Autodesk Fusion 360 part; units mm, degrees
(part 5 of 5)
  line L479 (14.0888, 19.1801) -> (13.1993, 20.0782)
  spline S498 degree 3 poles (13.1993, 20.0782) (12.7098, 20.5721) (12.0642, 21.2311) (11.7643, 21.5427) knots 0 0 0 0 1 1 1 1
  spline S499 degree 3 poles (11.7643, 21.5427) (11.0509, 22.2836) (10.6839, 22.4136) (10.1068, 22.1302) knots 0 0 0 0 1 1 1 1
  spline S500 degree 3 poles (10.1068, 22.1302) (9.2919, 21.7302) (9.2967, 20.4435) (10.115, 20.0204) knots 0 0 0 0 1 1 1 1
  spline S501 degree 3 poles (10.115, 20.0204) (10.2289, 19.9616) (10.2292, 19.9609) (10.2292, 19.6142) knots 0 0 0 0 1 1 1 1
  line L480 (10.2292, 19.6142) -> (10.2292, 19.2671)
  line L481 (10.2292, 19.2671) -> (10.124, 19.2919)
  spline S502 degree 3 poles (10.124, 19.2919) (9.1475, 19.5213) (8.5366, 20.6684) (8.8609, 21.6642) knots 0 0 0 0 1 1 1 1
  spline S503 degree 3 poles (8.7977, 26.7455) (8.8953, 27.5059) (9.4553, 28.1595) (10.2653, 28.4591) knots 0 0 0 0 1 1 1 1
  spline S504 degree 3 poles (10.2653, 28.4591) (10.5632, 28.5691) (12.2025, 28.6032) (12.6135, 28.5076) knots 0 0 0 0 1 1 1 1
  spline S505 degree 3 poles (12.6135, 28.5076) (14.8462, 27.9885) (14.8204, 24.7336) (12.5795, 24.2631) knots 0 0 0 0 1 1 1 1
  spline S506 degree 3 poles (12.5795, 24.2631) (12.2114, 24.1857) (10.8463, 24.1854) (10.4824, 24.2624) knots 0 0 0 0 1 1 1 1
  spline S507 degree 3 poles (10.4824, 24.2624) (9.5743, 24.455) (8.8991, 25.1822) (8.7787, 26.0974) knots 0 0 0 0 1 1 1 1
  spline S508 degree 3 poles (8.7787, 26.0974) (8.7488, 26.3241) (8.7505, 26.376) (8.7977, 26.7455) knots 0 0 0 0 1 1 1 1
  spline S509 degree 3 poles (8.8609, 32.4032) (9.1953, 33.4296) (10.3726, 33.9445) (11.3178, 33.4774) knots 0 0 0 0 1 1 1 1
  spline S510 degree 3 poles (11.3178, 33.4774) (11.5782, 33.3484) (11.7144, 33.2339) (12.4391, 32.5326) knots 0 0 0 0 1 1 1 1
  spline S511 degree 3 poles (12.4391, 32.5326) (13.0246, 31.9664) (13.2898, 31.7346) (13.352, 31.7346) knots 0 0 0 0 1 1 1 1
  line L482 (13.352, 31.7346) -> (13.4394, 31.7346)
  line L483 (13.4394, 31.7346) -> (13.4394, 32.6897)
  line L484 (13.4394, 32.6897) -> (13.4394, 33.6453)
  line L485 (13.4394, 33.6453) -> (13.7641, 33.6453)
  line L486 (13.7641, 33.6453) -> (14.0891, 33.6453)
  line L487 (14.0891, 33.6453) -> (14.0888, 31.782)
  line L488 (14.0888, 31.782) -> (14.0888, 29.9192)
  line L489 (14.0888, 29.9192) -> (13.2182, 30.798)
  spline S512 degree 3 poles (13.2182, 30.798) (12.7398, 31.2816) (12.0938, 31.9406) (11.7829, 32.2629) knots 0 0 0 0 1 1 1 1
  spline S513 degree 3 poles (11.7829, 32.2629) (11.0485, 33.0244) (10.6881, 33.1548) (10.1068, 32.8693) knots 0 0 0 0 1 1 1 1
  spline S514 degree 3 poles (10.1068, 32.8693) (9.2919, 32.4696) (9.2967, 31.1825) (10.115, 30.7594) knots 0 0 0 0 1 1 1 1
  spline S515 degree 3 poles (10.115, 30.7594) (10.2289, 30.7006) (10.2292, 30.7003) (10.2292, 30.3536) knots 0 0 0 0 1 1 1 1
  line L490 (10.2292, 30.3536) -> (10.2292, 30.0062)
  line L491 (10.2292, 30.0062) -> (10.124, 30.0309)
  spline S516 degree 3 poles (10.124, 30.0309) (9.1502, 30.2583) (8.5373, 31.4095) (8.8609, 32.4032) knots 0 0 0 0 1 1 1 1
  spline S517 degree 3 poles (8.8541, 37.2252) (9.1798, 38.1762) (10.3131, 38.4655) (10.9852, 37.769) knots 0 0 0 0 1 1 1 1
  spline S518 degree 3 poles (10.9852, 37.769) (11.2074, 37.5389) (11.2642, 37.5365) (11.4121, 37.7514) knots 0 0 0 0 1 1 1 1
  spline S519 degree 3 poles (11.4121, 37.7514) (12.1451, 38.8167) (13.8064, 38.4858) (14.2081, 37.1949) knots 0 0 0 0 1 1 1 1
  spline S520 degree 3 poles (14.2081, 37.1949) (14.5301, 36.1603) (13.9237, 35.1267) (12.855, 34.8897) knots 0 0 0 0 1 1 1 1
  line L492 (12.855, 34.8897) -> (12.7484, 34.866)
  line L493 (12.7484, 34.866) -> (12.7594, 35.1993)
  line L494 (12.7594, 35.1993) -> (12.7707, 35.5326)
  line L495 (12.7707, 35.5326) -> (12.9007, 35.5659)
  spline S521 degree 3 poles (12.9007, 35.5659) (13.6213, 35.7524) (13.858, 36.9373) (13.288, 37.5072) knots 0 0 0 0 1 1 1 1
  spline S522 degree 3 poles (13.288, 37.5072) (12.7181, 38.0772) (11.8173, 37.716) (11.7313, 36.8826) knots 0 0 0 0 1 1 1 1
  line L496 (11.7313, 36.8826) -> (11.7089, 36.6645)
  line L497 (11.7089, 36.6645) -> (11.354, 36.6645)
  line L498 (11.354, 36.6645) -> (10.999, 36.6645)
  line L499 (10.999, 36.6645) -> (10.9546, 36.8771)
  spline S523 degree 3 poles (10.9546, 36.8771) (10.7974, 37.6355) (9.6995, 37.6974) (9.4997, 36.959) knots 0 0 0 0 1 1 1 1
  spline S524 degree 3 poles (9.4997, 36.959) (9.3924, 36.5624) (9.5282, 36.1696) (9.8275, 36.0107) knots 0 0 0 0 1 1 1 1
  line L500 (9.8275, 36.0107) -> (9.9998, 35.9195)
  line L501 (9.9998, 35.9195) -> (9.9998, 35.5807)
  line L502 (9.9998, 35.5807) -> (9.9998, 35.2423)
  line L503 (9.9998, 35.2423) -> (9.8945, 35.2677)
  spline S525 degree 3 poles (9.8945, 35.2677) (9.0415, 35.4762) (8.5634, 36.3756) (8.8541, 37.2252) knots 0 0 0 0 1 1 1 1
  spline S526 degree 3 poles (9.5551, 25.8845) (9.661, 25.4921) (9.9492, 25.1581) (10.3393, 24.9751) knots 0 0 0 0 1 1 1 1
  line L504 (10.3393, 24.9751) -> (10.5539, 24.8743)
  line L505 (10.5539, 24.8743) -> (11.5476, 24.8743)
  spline S527 degree 3 poles (11.5476, 24.8743) (12.4914, 24.8743) (12.5502, 24.8785) (12.7215, 24.9586) knots 0 0 0 0 1 1 1 1
  spline S528 degree 3 poles (12.7215, 24.9586) (13.9292, 25.5217) (13.8026, 27.4905) (12.5351, 27.8588) knots 0 0 0 0 1 1 1 1
  spline S529 degree 3 poles (12.5351, 27.8588) (12.2001, 27.9562) (10.6189, 27.9208) (10.3819, 27.8104) knots 0 0 0 0 1 1 1 1
  spline S530 degree 3 poles (10.3819, 27.8104) (9.6772, 27.4819) (9.3377, 26.6911) (9.5551, 25.8845) knots 0 0 0 0 1 1 1 1
  spline S531 degree 3 poles (9.8687, 26.7764) (9.952, 27.0199) (10.189, 27.2758) (10.4504, 27.4041) knots 0 0 0 0 1 1 1 1
  line L506 (10.4504, 27.4041) -> (10.6684, 27.5115)
  line L507 (10.6684, 27.5115) -> (11.5283, 27.5115)
  spline S532 degree 3 poles (11.5283, 27.5115) (12.3528, 27.5115) (12.3968, 27.5077) (12.5901, 27.4203) knots 0 0 0 0 1 1 1 1
  spline S533 degree 3 poles (12.5901, 27.4203) (13.4579, 27.0282) (13.4652, 25.737) (12.6018, 25.3376) knots 0 0 0 0 1 1 1 1
  spline S534 degree 3 poles (12.6018, 25.3376) (12.3528, 25.2224) (10.9175, 25.1942) (10.5869, 25.2981) knots 0 0 0 0 1 1 1 1
  spline S535 degree 3 poles (10.5869, 25.2981) (9.9853, 25.4873) (9.6589, 26.1597) (9.8687, 26.7764) knots 0 0 0 0 1 1 1 1
  spline S536 degree 3 poles (10.0792, -35.4233) (10.1329, -35.5155) (10.3296, -35.5117) (10.3802, -35.4174) knots 0 0 0 0 1 1 1 1
  spline S537 degree 3 poles (10.3802, -35.4174) (10.428, -35.3277) (13.039, 14.4139) (13.0029, 14.5566) knots 0 0 0 0 1 1 1 1
  spline S538 degree 3 poles (13.0029, 14.5566) (12.9891, 14.6123) (12.9362, 14.6994) (12.8853, 14.7499) knots 0 0 0 0 1 1 1 1
  line L508 (12.8853, 14.7499) -> (12.7931, 14.8421)
  line L509 (12.7931, 14.8421) -> (11.5469, 14.8421)
  spline S539 degree 3 poles (11.5469, 14.8421) (10.221, 14.8421) (10.1921, 14.8383) (10.0958, 14.6519) knots 0 0 0 0 1 1 1 1
  spline S540 degree 3 poles (10.0958, 14.6519) (10.0246, 14.5143) (10.008, -35.3012) (10.0792, -35.4233) knots 0 0 0 0 1 1 1 1
  spline S541 degree 3 poles (10.0975, 42.9235) (10.1941, 42.7457) (10.2306, 42.7412) (11.5469, 42.7412) knots 0 0 0 0 1 1 1 1
  line L510 (11.5469, 42.7412) -> (12.7931, 42.7412)
  line L511 (12.7931, 42.7412) -> (12.8853, 42.8334)
  spline S542 degree 3 poles (12.8853, 42.8334) (12.9362, 42.884) (12.9891, 42.971) (13.0029, 43.0267) knots 0 0 0 0 1 1 1 1
  spline S543 degree 3 poles (13.0029, 43.0267) (13.039, 43.1695) (10.428, 92.911) (10.3802, 93.0008) knots 0 0 0 0 1 1 1 1
  spline S544 degree 3 poles (10.3802, 93.0008) (10.3272, 93.0995) (10.1305, 93.0988) (10.0775, 92.9997) knots 0 0 0 0 1 1 1 1
  spline S545 degree 3 poles (10.0775, 92.9997) (10.007, 92.8677) (10.027, 43.0539) (10.0975, 42.9235) knots 0 0 0 0 1 1 1 1
extrude "Extrude31" add sketch "Sketch17" along normal blind 2.3813 contours S368 S369 S370 | S371 S372 S373 | S374 L246 L247 L248 L249 S375 S376 S377 L250 L251 L252 L253 S378 S379 | S380 S381 L254 L255 S382 S383 S384 S385 S386 S387 L256 L257 L258 L259 S388 S389 S390 S391 | S403 S404 S405 S406 S407 S408 L326 L327 L328 L329 L330 L331 L332 L333 L334 L335 L336 L337 S409 | S410 S411 S412 S413 L338 L339 L340 L341 L342 L343 | L344 L345 L346 L347 L348 L349 L350 L351 L352 L353 L354 L355 L356 L357 L358 L359 | L360 L361 L362 L363 L364 L365 L366 L367
extrude "Extrude32" add sketch "Sketch17" along normal blind 1.5875 contours S307 S308 S309 S310 | S311 S312 S313 S314 | S315 S316 S317 S318 L124 L125 S319 S320 L126 L127 S321 L128 L129 S322 S323 | S324 S325 S326 S327 L130 L131 L132 L133 S328 S329 S330 S331 S332 L134 L135 L136 L137 S333 | L198 L199 L200 L201 L202 L203 L204 L205 S345 S346 S347 S348 S349 S350 S351 L206 L207 | L208 L209 S352 S353 L210 L211 S354 S355 L212 L213 | L214 L215 L216 L217 L218 L219 L220 L221 L222 L223 L224 L225 L226 L227 L228 L229 | L230 L231 L232 L233 L234 L235 L236 L237 | S422 S423 S424 S425 | S426 S427 S428 S429 | L376 L377 L378 L379 S431 L380 L381 L382 L383 | L390 L391 L392 L393 S434 S435 L394 L395 | L420 L421 L422 L423 S461 L424 L425 L426 L427
extrude "Extrude33" add sketch "Sketch16" along normal blind 1.5875 contours S386 S387 S388 S389 | S390 S391 S392 S393 | L323 L324 L325 L326 S402 L327 L328 L329 L330 | L339 L340 L341 L342 S404 S405 L343 L344 | L367 L368 L369 L370 S432 L371 L372 L373 L374
extrude "Extrude4" [suppressed]
extrude "Extrude5" [suppressed]
extrude "Extrude6" [suppressed]
extrude "Extrude1" [suppressed]
equation "d22 = d20"
equation "d55 = d54"
equation "d56 = d54"
equation "d57 = d54"
equation "d68 = d67"
